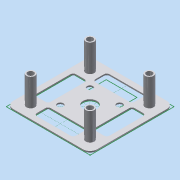
# Autodesk Inventor part: SensorMount_bottom
Saved by Autodesk Inventor 2015 (Build 190159000, 159)
## iProperties
Created: 2015-08-15
Part Number: SensorMount_bottom
Material: Aluminum 6061
Document SubType Name: Modeling
Designer: Raphael
Density: 2.71 g/cm^3
Appearance: Aluminum - Flat
Author: Raphael
Autodesk Inventor part; units mm, degrees
ref_plane "YZ Plane Vertical Spine" through (0, 0, 0) normal (1, 0, 0) x (0, 1, 0)
ref_plane "XZ Plane Horizontal" through (0, 0, 0) normal (0, 1, 0) x (-1, 0, 0)
ref_plane "XY Plane Vertical Span" through (0, 0, 0) normal (0, 0, 1) x (1, 0, 0)
derived "SensorMount_top.ipt"
sketch "Sketch1" plane through (0, 0, 0) normal (0, 1, 0) x (-1, 0, 0)
  line L0 (0, 0) -> (60, 0)
  line L1 (60, 0) -> (60, -60)
  line L2 (60, -60) -> (0, -60)
  line L3 (0, -60) -> (0, 0)
  circle A0 centre (51.2132, -8.7868) radius 2.15
  circle A1 centre (8.7868, -51.2132) radius 2.15
  circle A2 centre (8.7868, -8.7868) radius 2.15
  circle A3 centre (51.2132, -51.2132) radius 2.15
  line L4 (51.2132, -8.7868) -> (8.7868, -51.2132) construction
  line L5 (51.2132, -51.2132) -> (8.7868, -8.7868) construction
  line L6 (51.2132, -8.7868) -> (8.7868, -8.7868) construction
  line L7 (21, -24.5) -> (39, -24.5) construction
  line L8 (39, -24.5) -> (39, -35.5) construction
  line L9 (39, -35.5) -> (21, -35.5) construction
  line L10 (21, -35.5) -> (21, -24.5) construction
  line L11 (30, 0) -> (30, -60) construction
  circle A4 centre (21, -24.5) radius 1.5
  circle A5 centre (21, -35.5) radius 1.5
  line L12 (19, -22.5) -> (41, -22.5) construction
  line L13 (41, -22.5) -> (41, -52.5) construction
  line L14 (41, -52.5) -> (19, -52.5) construction
  line L15 (19, -52.5) -> (19, -22.5) construction
  line L16 (21, -24.5) -> (19, -24.5) construction
  line L17 (21, -24.5) -> (21, -22.5) construction
  line L18 (39, -24.5) -> (41, -24.5) construction
  circle A6 centre (39, -24.5) radius 1.5
  circle A7 centre (39, -35.5) radius 1.5
  arc A8 (25, -30) -> (35, -30) centre (30, -30) ccw
  line L19 (19, -52.5) -> (41, -52.5)
  line L20 (41, -52.5) -> (41, -38.5196)
  line L21 (41, -38.5196) -> (19, -38.5196)
  line L22 (19, -38.5196) -> (19, -52.5)
  circle A9 centre (21, -24.5) radius 2.25
  circle A10 centre (21, -35.5) radius 2.25
  circle A11 centre (39, -24.5) radius 2.25
  circle A12 centre (39, -35.5) radius 2.25
  line L23 (25, -30) -> (35, -30) construction
  line L24 (35, -30) -> (35, -23)
  line L25 (35, -23) -> (25, -23)
  line L26 (25, -23) -> (25, -30)
  line L27 (40.5, -26.1771) -> (40.5, -33.8229)
  line L28 (37.5, -33.8229) -> (37.5, -26.1771)
  line L29 (4, -16) -> (14, -16)
  line L30 (14, -16) -> (14, -44)
  line L31 (14, -44) -> (4, -44)
  line L32 (4, -44) -> (4, -16)
  line L33 (16, -4) -> (44, -4)
  line L34 (44, -4) -> (44, -14)
  line L35 (44, -14) -> (16, -14)
  line L36 (16, -14) -> (16, -4)
  line L37 (46, -44) -> (56, -44)
  line L38 (46, -16) -> (46, -44)
  line L39 (56, -44) -> (56, -16)
  line L40 (56, -16) -> (46, -16)
  point P0 (60, -30)
  point P1 (39, -30)
  point P2 (30, -24.5)
sketch "Sketch3" plane through (0, 0, 0) normal (0, 1, 0) x (-1, 0, 0)
  line L0 (0, 0) -> (60, 0) projected
  line L1 (60, 0) -> (60, -60) projected
  line L2 (60, -60) -> (0, -60) projected
  line L3 (0, -60) -> (0, 0) projected
  circle A0 centre (8.7868, -51.2132) radius 2.15 projected
  circle A1 centre (8.7868, -8.7868) radius 2.15 projected
  circle A2 centre (51.2132, -8.7868) radius 2.15 projected
  circle A3 centre (51.2132, -51.2132) radius 2.15 projected
  line L4 (60, 0) -> (60, -60)
  line L5 (0, -60) -> (0, 0)
  line L6 (60, 0) -> (0, 0)
  line L7 (60, -60) -> (0, -60)
  circle A4 centre (51.2132, -8.7868) radius 2.15
  circle A5 centre (51.2132, -51.2132) radius 2.15
  circle A6 centre (8.7868, -51.2132) radius 2.15
  circle A7 centre (8.7868, -8.7868) radius 2.15
  line L8 (51.2132, -51.2132) -> (8.7868, -8.7868) construction
  line L9 (51.2132, -8.7868) -> (8.7868, -51.2132) construction
  circle A8 centre (19.3934, -19.3934) radius 2.15
  circle A9 centre (19.3934, -40.6066) radius 2.15
  circle A10 centre (40.6066, -40.6066) radius 2.15
  circle A11 centre (40.6066, -19.3934) radius 2.15
  circle A12 centre (51.2132, -8.7868) radius 3
  circle A13 centre (8.7868, -8.7868) radius 3
  circle A14 centre (8.7868, -51.2132) radius 3
  circle A15 centre (51.2132, -51.2132) radius 3
  circle A16 centre (30, -30) radius 5
  line L10 (46, -16) -> (46, -44) projected
  line L11 (46, -44) -> (56, -44) projected
  line L12 (56, -44) -> (56, -16) projected
  line L13 (56, -16) -> (46, -16) projected
  line L14 (16, -4) -> (44, -4) projected
  line L15 (44, -4) -> (44, -14) projected
  line L16 (44, -14) -> (16, -14) projected
  line L17 (16, -14) -> (16, -4) projected
  line L18 (14, -16) -> (14, -44) projected
  line L19 (4, -16) -> (14, -16) projected
  line L20 (4, -44) -> (4, -16) projected
  line L21 (14, -44) -> (4, -44) projected
  line L22 (25, -30) -> (35, -30) construction
  line L23 (16, -56) -> (44, -56)
  line L24 (44, -56) -> (44, -46)
  line L25 (44, -46) -> (16, -46)
  line L26 (16, -46) -> (16, -56)
  dimension "d3" = 4.3
  dimension "d4" = 4.3
  dimension "d5" = 4.3
  dimension "d6" = 4.3
  dimension "d7" = 30
  dimension "d8" = 30
  dimension "d9" = 6
  dimension "d10" = 6
  dimension "d11" = 6
  dimension "d12" = 6
  dimension "d17" = 10
  constraints: 16 end point, 13 centre point, 8 coincident, 4 concentric, 4 point on line, 4 symmetric about line, 3 equal length, 1 horizontal, 1 horizontal alignment, 1 midpoint, 1 vertical alignment
  measures "d3" diameter of A8
  measures "d4" diameter of A9
  measures "d5" diameter of A10
  measures "d6" diameter of A11
  measures "d7" distance of A10.centre A8.centre
  measures "d8" distance of A9.centre A11.centre
  measures "d9" diameter of A12
  measures "d10" diameter of A13
  measures "d11" diameter of A14
  measures "d12" diameter of A15
  measures "d17" diameter of A16
extrude "Extrusion1" add sketch "Sketch3" along normal blind 1 contours L0 L1 L2 L3
extrude "Extrusion2" add sketch "Sketch3" along normal blind 20.5 contours A12 | A13 | A14 | A15
fillet "Fillet1" radius 5 4 edges at (0, 0.5, 0) (0, 0.5, -60) (-60, 0.5, 0) (-60, 0.5, -60)
fillet "Fillet2" radius 2 16 edges at (-44, 0.5, -46) (-44, 0.5, -56) (-56, 0.5, -44) (-44, 0.5, -14) (-14, 0.5, -44) (-46, 0.5, -44) (-16, 0.5, -56) (-16, 0.5, -14) (-4, 0.5, -44) (-4, 0.5, -16) (-16, 0.5, -46) (-16, 0.5, -4) (-46, 0.5, -16) (-14, 0.5, -16) (-44, 0.5, -4) (-56, 0.5, -16)
body "Solid2"
